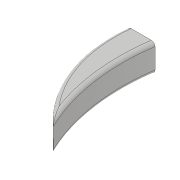
# Autodesk Inventor part: dog tail 3
Saved by Autodesk Inventor 2019 (Build 230136000, 136)
## iProperties
Created: 2019-10-12
Part Number: dog tail 3
Material: Generic
Document SubType Name: Modeling
Designer: Lenovo
Density: 1 g/cm^3
Appearance: Default
Author: Lenovo
Autodesk Inventor part; units mm, degrees
ref_plane "YZ Plane" through (0, 0, 0) normal (1, 0, 0) x (0, 1, 0)
ref_plane "XZ Plane" through (0, 0, 0) normal (0, 1, 0) x (-1, 0, 0)
ref_plane "XY Plane" through (0, 0, 0) normal (0, 0, 1) x (1, 0, 0)
sketch "Sketch1" plane through (0, 0, 0) normal (0, 1, 0) x (-1, 0, 0)
  line L0 (0.6302, -4.8681) -> (15.6302, -4.8681)
  arc A0 (15.6302, -4.8681) -> (-9.3835, 60.5102) centre (-60.6026, 3.4395) ccw
  arc A1 (0.6302, -4.8681) -> (-9.3835, 60.5102) centre (-111.0302, 11.4854) ccw
  point P0 (0, 0)
  dimension "d0" = 15
  dimension "d1" = 70
  constraints: 4 point on circle, 2 centre point, 2 end point, 1 horizontal
  measures "d0" distance of L0.start L0.end
  measures "d1" distance of L0.end A0.end
extrude "Extrusion1" add sketch "Sketch1" along normal blind 15
fillet "Fillet1" radius 2 4 edges at (-0.5205, 15, 28.5711) (-0.5205, 0, 28.5711) (-11.0185, 15, 30.8417) (-11.0185, 0, 30.8417)
body "Solid1"
